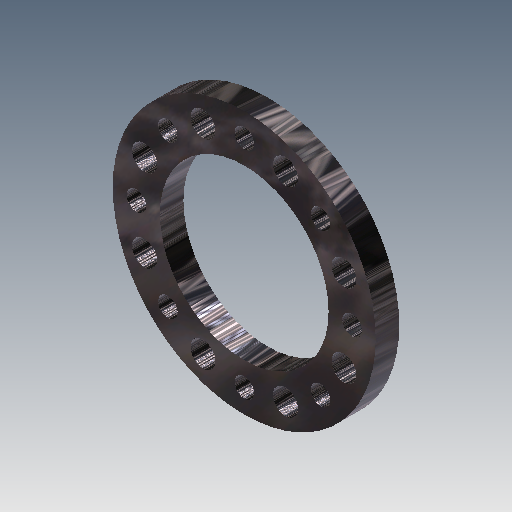
# Autodesk Inventor part: 出力部品B_ダブルスラスト用(t2_アルミ)
Saved by Autodesk Inventor 2019.4 (Build 234330000, 330)
## iProperties
Created: 2018-08-09
Part Number: 出力部品B_ダブルスラスト用(t2_アルミ)
Material: アルミニウム 6061
Document SubType Name: Modeling
Designer: Owner
Mass: 3.3595 g
Surface Area: 17.7764 cm^2
Volume: 1.24426 cm^3
Density: 2.7 g/cm^3
Appearance: アルミニウム - フラット
Author: Owner
Autodesk Inventor part; units mm, degrees
ref_plane "YZ Plane" through (0, 0, 0) normal (1, 0, 0) x (0, 1, 0)
ref_plane "XZ Plane" through (0, 0, 0) normal (0, 1, 0) x (-1, 0, 0)
ref_plane "XY Plane" through (0, 0, 0) normal (0, 0, 1) x (1, 0, 0)
sketch "スケッチ1" plane through (0, 0, 0) normal (0, 0, 1) x (1, 0, 0)
  circle A0 centre (0, 0) radius 15.5 construction
  circle A1 centre (-16.7262, 17.2115) radius 1.6 projected
  circle A2 centre (0.3431, 23.9975) radius 1.6 projected
  circle A3 centre (17.2115, 16.7262) radius 1.6 projected
  circle A4 centre (23.9975, -0.3431) radius 1.6 projected
  circle A5 centre (16.7262, -17.2115) radius 1.6 projected
  circle A6 centre (-0.3431, -23.9975) radius 1.6 projected
  circle A7 centre (-17.2115, -16.7262) radius 1.6 projected
  circle A8 centre (-23.9975, 0.3431) radius 1.6 projected
  circle A9 centre (0, 0) radius 27.5 projected
  circle A10 centre (0, 0) radius 5.1 projected
  circle A11 centre (4.9497, -4.9497) radius 1.1 projected
  circle A12 centre (7, 0) radius 1.1 projected
  circle A13 centre (4.9497, 4.9497) radius 1.1 projected
  circle A14 centre (0, 7) radius 1.1 projected
  circle A15 centre (-4.9497, 4.9497) radius 1.1 projected
  circle A16 centre (-7, 0) radius 1.1 projected
  circle A17 centre (-4.9497, -4.9497) radius 1.1 projected
  circle A18 centre (0, -7) radius 1.1 projected
  circle A19 centre (0, 0) radius 20.5 projected
  circle A20 centre (0, 0) radius 10.75
  line L0 (0, 0) -> (13.125, 0) construction
  line L1 (9.2808, -9.2808) -> (0, 0) construction
  line L2 (0, 0) -> (12.7033, -5.2619) construction
  circle A21 centre (12.7033, -5.2619) radius 1.6
  circle A22 centre (0, 0) radius 16.75
  line L3 (0, 0) -> (0, -8.1)
  line L4 (0, -10.75) -> (0, -16.75)
  circle A23 centre (0, 0) radius 13.75 construction
  circle A24 centre (12.7033, 5.2619) radius 1.6
  circle A25 centre (0, 0) radius 13.75 construction
  circle A26 centre (5.2619, 12.7033) radius 1.6
  circle A27 centre (0, 0) radius 13.75 construction
  circle A28 centre (-5.2619, 12.7033) radius 1.6
  circle A29 centre (0, 0) radius 13.75 construction
  circle A30 centre (-12.7033, 5.2619) radius 1.6
  circle A31 centre (0, 0) radius 13.75 construction
  circle A32 centre (-12.7033, -5.2619) radius 1.6
  circle A33 centre (0, 0) radius 13.75 construction
  circle A34 centre (-5.2619, -12.7033) radius 1.6
  circle A35 centre (0, 0) radius 13.75 construction
  circle A36 centre (5.2619, -12.7033) radius 1.6
  circle A37 centre (0, 0) radius 13.75 construction
  dimension "d14" = 21.5
  dimension "d15" = 33.5
  dimension "d0" = 13.75
  dimension "d1" = 22.5
  dimension "d2" = 3.2
  dimension "d18" = 27.5
  dimension "d21" = 360
  constraints: 16 centre point, 10 end point, 4 coincident, 3 vertical alignment, 2 vertical, 1 horizontal, 38 other
  measures "d0" distance of L0.start L2.end
  measures "d1" angle of L0 L2
  measures "d2" diameter of A21
  measures "d18" diameter of A23
extrude "押し出し3" add sketch "スケッチ1" along normal blind 3 contours A22
sketch "スケッチ2" plane through (0, 0, 3) normal (0, 0, 1) x (1, 0, 0)
  circle A0 centre (0, 0) radius 16.75
  circle A1 centre (5.2619, -12.7033) radius 1.6 projected
  circle A2 centre (0, 0) radius 13.75 construction
  line L0 (0, 0) -> (5.2619, -12.7033)
  line L1 (0, 0) -> (-5.2619, -12.7033)
  line L2 (0, -13.75) -> (0, 0) construction
  circle A3 centre (0, -13.75) radius 1.25
  circle A4 centre (9.7227, -9.7227) radius 1.25
  circle A5 centre (13.75, 0) radius 1.25
  circle A6 centre (9.7227, 9.7227) radius 1.25
  circle A7 centre (0, 13.75) radius 1.25
  circle A8 centre (-9.7227, 9.7227) radius 1.25
  circle A9 centre (-13.75, 0) radius 1.25
  circle A10 centre (-9.7227, -9.7227) radius 1.25
  dimension "d25" = 2.5
  dimension "d28" = 360
  constraints: 10 centre point, 6 end point, 3 coincident, 3 point on circle, 1 vertical, 17 other
  measures "d25" diameter of A3
extrude "押し出し4" cut sketch "スケッチ2" against normal through all contours A3 | A4 | A5 | A6 | A7 | A8 | A9 | A10
